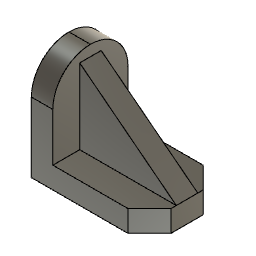
Figure A1 v1 (Autodesk Fusion 360 design; units mm, degrees)
Autodesk Fusion 360 part; units mm, degrees
note: some values were not read from the file. Set by a fixed rule: which sketch regions a step uses.
sketch "Sketch1" plane through (0, 0, 0) normal (0, 0, 1) x (1, 0, 0)
sketch "Sketch3" plane through (0, 0, 0) normal (0, 0, 1) x (1, 0, 0)
  line L0 (0, 0) -> (66, 0)
  line L1 (66, 0) -> (66, 42)
  line L2 (66, 42) -> (0, 42)
  line L3 (0, 42) -> (0, 0)
  line L4 (66, 0) -> (54, 0)
  line L5 (54, 0) -> (54, 12)
  line L6 (54, 12) -> (66, 12)
  line L7 (66, 12) -> (66, 0)
  line L8 (66, 42) -> (54, 42)
  line L9 (54, 42) -> (54, 30)
  line L10 (54, 30) -> (66, 30)
  line L11 (66, 30) -> (66, 42)
  line L12 (54, 42) -> (66, 30)
  line L13 (66, 12) -> (54, 0)
  point P0 (54, 42)
  point P1 (66, 30)
  point P2 (54, 0)
  point P3 (66, 12)
  dimension "d11" = 66
  dimension "d12" = 42
  dimension "d13" = 12
  dimension "d14" = 12
  dimension "d15" = 12
  dimension "d16" = 12
  constraint horizontal L0
  constraint vertical L1
  constraint horizontal L2
  constraint vertical L3
  constraint coincident L0.start L3.end
  constraint horizontal L4
  constraint vertical L5
  constraint horizontal L6
  constraint vertical L7
  constraint horizontal L8
  constraint vertical L9
  constraint horizontal L10
  constraint vertical L11
  constraint coincident P0 L8.end
  constraint coincident P1 L10.end
  constraint coincident P2 L4.end
  constraint coincident P3 L6.end
  measures "d11" distance of L0.start L0.end
  measures "d12" distance of L0.start L2.end
  measures "d13" distance of L0.end L4.end
  measures "d14" distance of L0.end P3
  measures "d15" distance of L1.end P0
  measures "d16" distance of L1.end P1
extrude "Extrude1" add sketch "Sketch3" along normal blind 12 contours L0 L1 L2 L3 L5 L6 L9 L10 | L5 L6 L13 | L9 L10 L12
sketch "Sketch4" plane through (0, 0, 0) normal (1, 0, 0) x (0, 1, 0)
  line L0 (0, 0) -> (42, 0)
  line L1 (42, 0) -> (42, 39)
  line L2 (21.0001, 60) -> (21, 60)
  line L3 (0, 39) -> (0, 0)
  line L4 (21, 0) -> (21, 39)
  line L5 (0, 39) -> (42, 39)
  arc A0 (21, 60) -> (0, 39) centre (21, 39) ccw
  arc A1 (42, 39) -> (21.0001, 60) centre (21, 39) ccw
  point P0 (0, 60)
  dimension "d19" = 42
  dimension "d20" = 60
  dimension "d21" = 39
  dimension "d22" = 21
  constraint horizontal L0
  constraint vertical L1
  constraint vertical L3
  constraint coincident L0.start L3.end
  constraint coincident L0 L4.start
  constraint perpendicular L0 L4
  constraint midpoint L0 L4.start
  constraint coincident L3 L5.start
  constraint coincident L1 L5.end
  constraint perpendicular L1 L5
  constraint coincident P0 L3
  constraint tangent L3 A0
  constraint tangent L1 A1
  constraint equal A0 A1
  measures "d19" distance of L0.start L0.end
  measures "d20" distance of L0.start P0
  measures "d21" distance of L4.start L4.end
  measures "d22" radius of A0
extrude "Extrude2" add sketch "Sketch4" along normal blind 12
sketch "Sketch5" plane through (0, 0, 12) normal (0, 0, 1) x (-1, 0, 0)
  line L0 (-12, -42) -> (-12, 0)
  line L1 (-12, 0) -> (-54, 0)
  line L2 (-54, 0) -> (-66, -12)
  line L3 (-66, -12) -> (-66, -30)
  line L4 (-66, -30) -> (-54, -42)
  line L5 (-54, -42) -> (-12, -42)
  line L6 (-25, 0) -> (-25, -15)
  line L7 (-25, -27) -> (-25, -42)
  line L8 (-25, -42) -> (-25, -27)
  line L9 (-12, -27) -> (-66, -27)
  line L10 (-66, -27) -> (-66, -15)
  line L11 (-66, -15) -> (-12, -15)
  line L12 (-12, -15) -> (-12, -27)
  dimension "d25" = 15
  dimension "d26" = 15
  dimension "d27" = 15
  dimension "d28" = 12
  constraint coincident L1 L6.start
  constraint perpendicular L1 L6
  constraint coincident L5 L7.end
  constraint perpendicular L5 L7
  constraint perpendicular L5 L8
  constraint horizontal L9
  constraint vertical L10
  constraint horizontal L11
  constraint vertical L12
  constraint coincident L0 L9.start
  measures "d25" distance of L7.end L7.start
  measures "d26" distance of L6.start L6.end
  measures "d27" distance of L6.start L6.end
  measures "d28" distance of L9.start L11.end
extrude "Extrude3" add sketch "Sketch5" along normal blind 42 contours L0 L3 L9 L10 L11 L12
sketch "Sketch6" plane through (0, 15, 0) normal (0, -1, 0) x (1, 0, 0)
  line L0 (12, 12) -> (66, 12)
  line L1 (66, 12) -> (66, 54)
  line L2 (66, 54) -> (12, 54)
  line L3 (12, 54) -> (12, 12)
  line L4 (66, 12) -> (12, 54)
  constraint coincident L0.end L1.start
  constraint coincident L2.end L3.start
extrude "Extrude4" cut sketch "Sketch6" against normal blind 29 contours L1 L2 L4
sketch "Sketch7" plane through (30.6923, 0, 39.4615) normal (0.613941, 0, 0.789352) x (0, 1, 0)
  line L0 (27, -44.73) -> (27, 23.6806)
  line L1 (27, 23.6806) -> (15, 23.6806)
  line L2 (15, 23.6806) -> (15, -44.73)
  line L3 (15, -44.73) -> (27, -44.73)
  dimension "d33" = 12
  measures "d33" distance of L0.end L1.end
sketch "Sketch2" plane through (0, 0, 0) normal (1, 0, 0) x (0, 1, 0)
  line L0 (0, 0) -> (42, 0)
  line L1 (42, 0) -> (42, 60)
  line L2 (42, 60) -> (0, 60)
  line L3 (0, 60) -> (0, 0)
  dimension "d5" = 60
  dimension "d6" = 42
  constraint horizontal L0
  constraint vertical L1
  constraint horizontal L2
  constraint vertical L3
  constraint coincident L0.start L3.end
  measures "d5" distance of L0.start L2.end
  measures "d6" distance of L1.end L2.end
